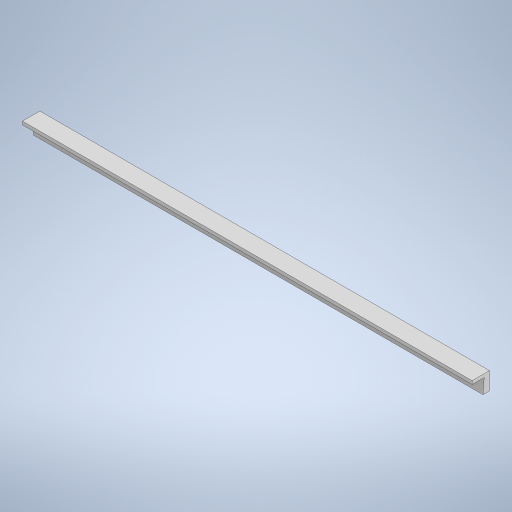
# Autodesk Inventor part: feederTrack_base
Saved by Autodesk Inventor 2024 (Build 280153000, 153)
## iProperties
Created: 2025-03-14
Part Number: feederTrack_base
Material: Generic
Document SubType Name: Modeling
Designer: simat
Density: 1 g/cm^3
Appearance: Default
Author: simat
Autodesk Inventor part; units mm, degrees
ref_plane "YZ Plane" through (0, 0, 0) normal (1, 0, 0) x (0, 1, 0)
ref_plane "XZ Plane" through (0, 0, 0) normal (0, 1, 0) x (-1, 0, 0)
ref_plane "XY Plane" through (0, 0, 0) normal (0, 0, 1) x (1, 0, 0)
sketch "Sketch1" plane through (0, 0, 0) normal (1, 0, 0) x (0, 1, 0)
  line L0 (0, -0.5091) -> (0, 1.2685)
  line L1 (0, 1.2685) -> (-0.3381, 1.2685)
  line L2 (-0.3381, 1.2685) -> (-0.3381, 0.0338)
  line L3 (-0.3381, 0.0338) -> (-1.794, 0.1577)
  line L4 (-1.794, 0.1577) -> (-1.794, -0.5091)
  line L5 (-1.794, -0.5091) -> (0, -0.5091)
  point P0 (0, 0)
  constraints: 12 end point, 3 perpendicular, 1 parallel, 1 vertical
extrude "Extrusion1" add sketch "Sketch1" along normal mid plane 45.9232
body "Solid1"
